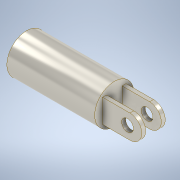
# Autodesk Inventor part: pistone
Saved by Autodesk Inventor 2022 (Build 260153000, 153)
## iProperties
Created: 2022-07-04
Part Number: pistone
Material: Titanio
Document SubType Name: Modeling
Designer: corra
Density: 4.51 g/cm^3
Appearance: Titanio
Mass: 25.6349 g
Surface Area: 23.9527 cm^2
Volume: 5.68402 cm^3
Author: corra
Autodesk Inventor part; units mm, degrees
ref_plane "YZ Plane" through (0, 0, 0) normal (1, 0, 0) x (0, 1, 0)
ref_plane "XZ Plane" through (0, 0, 0) normal (0, 1, 0) x (-1, 0, 0)
ref_plane "XY Plane" through (0, 0, 0) normal (0, 0, 1) x (1, 0, 0)
sketch "Schizzo1" plane through (0, 0, 0) normal (1, 0, 0) x (0, 1, 0)
  circle A0 centre (0, 0) radius 5
  dimension "d0" = 10
  constraints: 1 centre point, 1 coincident
  measures "d0" diameter of A0
extrude "Estrusione1" add sketch "Schizzo1" along normal blind 22.39
sketch "Schizzo2" plane through (22.39, 0, 0) normal (1, 0, 0) x (0, 0, -1)
  line L0 (-3, 3) -> (3, 3)
  line L1 (3, 3) -> (3, -3)
  line L2 (3, -3) -> (-3, -3)
  line L3 (-3, -3) -> (-3, 3)
  line L4 (-3, 3) -> (3, -3) construction
  line L5 (3, 3) -> (-3, -3) construction
  point P0 (0, 0)
  point P1 (0, 0)
  point P2 (0, 0)
  dimension "d3" = 6
  dimension "d4" = 6
  constraints: 12 end point, 3 midpoint, 2 parallel, 1 coincident, 1 horizontal, 1 perpendicular
  measures "d3" distance of L1.end L2.end
  measures "d4" distance of L0.end L1.end
extrude "Estrusione2" add sketch "Schizzo2" along normal blind 10
sketch "Schizzo5" plane through (22.39, 3, 3) normal (0, 1, 0) x (1, 0, 0)
  line L0 (0, -2) -> (0, 8) projected
  line L1 (10, 5) -> (0, 5)
  line L2 (0, 5) -> (0, 1)
  line L3 (0, 1) -> (10, 1)
  line L4 (10, 1) -> (10, 5)
  line L5 (10, 6) -> (10, 0) projected
  point P0 (-22.39, 3)
  point P1 (10, 3)
  point P2 (0, 5)
  dimension "d19" = 4
  constraints: 8 end point, 2 midpoint, 2 parallel, 1 horizontal, 1 perpendicular, 1 point on line
  measures "d19" distance between parallel lines of L1 L3
extrude "Estrusione5" cut sketch "Schizzo5" against normal blind 15
sketch "Schizzo6" plane through (22.39, -3, 3) normal (0, 0, 1) x (1, 0, 0)
  circle A0 centre (6.39, 3) radius 1.5
  line L0 (0, 0) -> (10, 0) projected
  line L1 (10, 6) -> (10, 0) projected
  line L2 (0, -2) -> (0, 8) projected
  point P0 (-22.39, 3)
  dimension "d22" = 3
  dimension "d24" = 3
  dimension "d28" = 6.39
  constraints: 1 centre point
  measures "d22" distance from line of L0 A0.centre
  measures "d24" diameter of A0
  measures "d28" distance from line of L2 A0.centre
extrude "Estrusione6" cut sketch "Schizzo6" against normal blind 15
fillet "Raccordo2" radius 3 4 edges at (32.39, 3, 2.5) (32.39, 3, -2.5) (32.39, -3, -2.5) (32.39, -3, 2.5)
